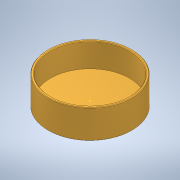
# Autodesk Inventor part: Shallow Dish
Saved by Autodesk Inventor 2021.1 (Build 251245010, 245A)
## iProperties
Created: 2025-09-16
Material: Brass, Soft Yellow
Document SubType Name: Modeling
Designer: SD
Density: 8.47 g/cm^3
Appearance: Brass - Satin
Mass: 14.6629 g
Surface Area: 26.1987 cm^2
Volume: 1.73115 cm^3
Project: Automatic Tea Steeping mechanism
Part Number: Shallow Dish
Length: 12.000 mm
BOM-Mass: 0.01466
BOM-Area: 0.003
Diameter: 35.000 mm
Author: SD
Title: Shallow Dish
Autodesk Inventor part; units mm, degrees
ref_plane "YZ Plane" through (0, 0, 0) normal (1, 0, 0) x (0, 1, 0)
ref_plane "XZ Plane" through (0, 0, 0) normal (0, 1, 0) x (-1, 0, 0)
ref_plane "XY Plane" through (0, 0, 0) normal (0, 0, 1) x (1, 0, 0)
sketch "Sketch4" plane through (0, 0, 0) normal (0, 1, 0) x (-1, 0, 0)
  circle A0 centre (0, 0) radius 17.5
  constraints: 1 centre point, 1 coincident, 1 other
extrude "Extrusion2" add sketch "Sketch4" along normal mid plane 12
sketch "Sketch12" plane through (0, 6, 0) normal (0, 1, 0) x (1, 0, 0)
  circle A0 centre (0, 0) radius 16.5
  dimension "d85" = 33
  constraints: 1 centre point, 1 coincident
  measures "d85" diameter of A0
extrude "Extrusion8" cut sketch "Sketch12" against normal blind 10
sketch "Sketch13" plane through (0, -4, 0) normal (0, 1, 0) x (1, 0, 0)
  point P0 (0, 0)
chamfer "Chamfer1" distance 0.2 angle 45 3 edges at (17.5, 6, 0) (-16.5, 6, 0) (17.5, -6, 0)
body "Solid2"
